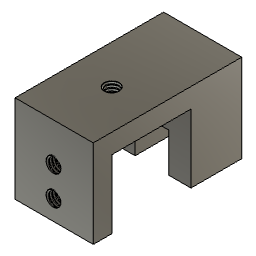
Slit Clip v2 (Autodesk Fusion 360 design; units mm, degrees)
Autodesk Fusion 360 part; units mm, degrees
sketch "Sketch1" plane through (0, 0, 0) normal (1, 0, 0) x (0, 1, 0) in component "Component"
  line L0 (0, 0) -> (13, 0)
  line L1 (0, 10) -> (13, 10)
  line L2 (13, 10) -> (13, 0)
  line L3 (0, 0) -> (0, 17.5)
  line L4 (0, 17.5) -> (-20, 17.5)
  line L5 (-20, 17.5) -> (-20, 0)
  line L6 (-20, 0) -> (-25, 0)
  line L7 (-25, 0) -> (-25, 22.5)
  line L8 (-25, 22.5) -> (13, 22.5)
  line L9 (13, 22.5) -> (13, 10)
  line L10 (-20, 17.5) -> (-20.2, 17.5)
  line L11 (-20.2, 17.5) -> (-20.2, 0)
  dimension "d1" = 13
  dimension "d2" = 17.5
  dimension "d3" = 20
  dimension "d4" = 22.5
  dimension "d5" = 0.2
  constraint coincident L0.start L3.start
  constraint horizontal L0
  constraint perpendicular L1 L3
  constraint perpendicular L3 L4
  constraint perpendicular L4 L5
  constraint perpendicular L5 L6
  constraint perpendicular L4 L7
  constraint perpendicular L7 L8
  constraint perpendicular L1 L9
  constraint horizontal L10
  constraint coincident L6 L11.end
  constraint perpendicular L6 L11
  measures "d1" distance of L0.start L0.end
  measures "d2" distance of L0.start L3.end
  measures "d3" distance of L3.end L4.end
  measures "d4" distance of L6.end L7.end
  measures "d5" distance of L4.end L10.end
extrude "Extrude1" add sketch "Sketch1" along normal mid plane 20 contours L0 L1 L2 L3 | L1 L3 L4 L6 L7 L8 L9 L10 L11 in component "Component"
extrude "Extrude2" cut sketch "Sketch1" along normal mid plane 8.6 contours L0 L1 L2 L3 in component "Component"
hole "Hole1" at (0, -10, 22.5) direction (0, 0, -1) diameter 3.416 depth 20 tip angle 118 in component "Component"
thread "Thread1" "ANSI Unified Screw Threads 0.164(#8) 8-32 UNC 2B" major diameter 4.1656 minor diameter 3.4163 pitch 0.7937 angle 60 modelled right hand crest width 0.2341 on face at (0.0851, -11.7059, 20.8333) crest through (1.7082, -10, 22.3016) in component "Component"
hole "Hole2" at (0, -25, 12.5) direction (0, 1, 0) diameter 3.416 depth 20 tip angle 118 in component "Component"
thread "Thread2" "ANSI Unified Screw Threads 0.164(#8) 8-32 UNC 2B" major diameter 4.1656 minor diameter 3.4163 pitch 0.7937 angle 60 modelled right hand crest width 0.2341 on face at (0.0851, -23.4, 10.7941) crest through (0, -24.8016, 10.7919) in component "Component"
hole "Hole3" at (0, -25, 5) direction (0, 1, 0) diameter 3.416 depth 20 tip angle 118 in component "Component"
thread "Thread3" "ANSI Unified Screw Threads 0.164(#8) 8-32 UNC 2B" major diameter 4.1656 minor diameter 3.4163 pitch 0.7937 angle 60 modelled right hand crest width 0.2341 on face at (0.0851, -23.4, 3.2941) crest through (0, -24.8016, 3.2918) in component "Component"
component "Component" placed x (1, 0, 0) y (0, 1, 0) z (0, 0, 1) at (0, 0, 0)
named bodies: "AS Slit Clip"
